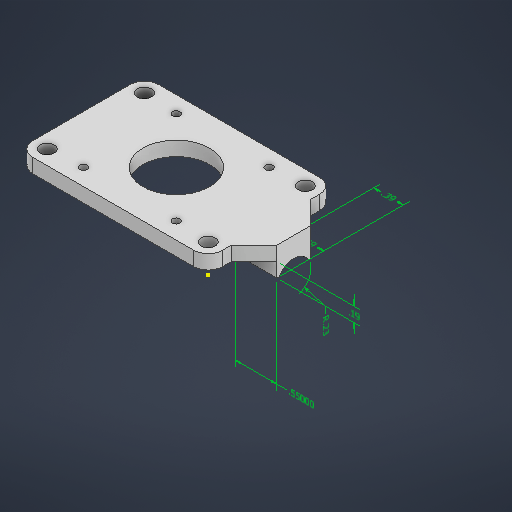
# Autodesk Inventor part: MotorTop
Saved by Autodesk Inventor 2026 (Build 300175000, 175)
## iProperties
Created: 2025-04-10
Part Number: MotorTop
Material: Generic
Document SubType Name: Modeling
Designer: jjgen
Density: 1 g/cm^3
Appearance: Default
Author: jjgen
## iProperties of the stored document MotorTop_3DPrint.ipt
Created: 2025-04-17
Part Number: MotorTop_3DPrint
Material: Generic
Document SubType Name: Modeling
Designer: sdcel
Density: 1 g/cm^3
Appearance: Default
Author: sdcel
Autodesk Inventor part; units mm, degrees
ref_plane "YZ Plane" through (0, 0, 0) normal (1, 0, 0) x (0, 1, 0)
ref_plane "XZ Plane" through (0, 0, 0) normal (0, 1, 0) x (-1, 0, 0)
ref_plane "XY Plane" through (0, 0, 0) normal (0, 0, 1) x (1, 0, 0)
sketch "Sketch1" plane through (0, 0, 0) normal (0, 1, 0) x (-1, 0, 0)
  line L0 (0, -4.826) -> (0, -37.338)
  line L1 (4.826, -42.164) -> (58.674, -42.164)
  line L2 (63.5, -37.338) -> (63.5, -4.826)
  line L3 (58.674, 0) -> (4.826, 0)
  arc A0 (4.826, 0) -> (0, -4.826) centre (4.826, -4.826) ccw
  arc A1 (63.5, -4.826) -> (58.674, 0) centre (58.674, -4.826) ccw
  arc A2 (58.674, -42.164) -> (63.5, -37.338) centre (58.674, -37.338) ccw
  arc A3 (0, -37.338) -> (4.826, -42.164) centre (4.826, -37.338) ccw
  circle A4 centre (4.826, -4.826) radius 4.826
  circle A5 centre (4.826, -37.338) radius 4.826
  circle A6 centre (58.674, -37.338) radius 4.826
  circle A7 centre (58.674, -4.826) radius 4.826
  circle A8 centre (58.674, -4.826) radius 2.3812
  circle A9 centre (58.674, -37.338) radius 2.3812
  circle A10 centre (4.826, -37.338) radius 2.3812
  circle A11 centre (4.826, -4.826) radius 2.3813
  point P0 (0, 0)
  point P1 (0, -42.164)
  point P2 (63.5, -42.164)
  dimension "d0" = 42.164
  dimension "d1" = 63.5
  dimension "d2" = 4.826
  dimension "d3" = 4.7625
  dimension "d4" = 4.7625
  dimension "d5" = 4.7625
  constraints: 10 centre point, 8 coincident, 8 end point, 8 point on circle, 8 tangent, 6 point on line, 5 equal radius, 3 perpendicular, 2 vertical alignment, 1 vertical, 4 other
  measures "d0" distance of point (0, 0) point (0, -42.164)
  measures "d1" distance of point (0, -42.164) point (63.5, -42.164)
  measures "d2" radius of A0
  measures "d3" diameter of A8
  measures "d4" diameter of A9
  measures "d5" diameter of A10
extrude "Extrusion1" add sketch "Sketch1" against normal blind 4.7625
sketch "Sketch2" plane through (0, -4.7625, 0) normal (0, -1, 0) x (1, 0, 0)
  line L0 (0, -37.338) -> (0, -4.826) projected
  line L1 (0, -21.082) -> (-63.5, -21.082)
  line L2 (-63.5, -4.826) -> (-63.5, -37.338) projected
  line L3 (-58.674, -42.164) -> (-4.826, -42.164) projected
  line L4 (-31.75, -42.164) -> (-31.75, 0)
  circle A0 centre (-31.75, -21.082) radius 11.176
  line L5 (-31.75, -21.082) -> (-16.2142, -5.5462)
  line L6 (-31.75, -21.082) -> (-9.779, -21.082) construction
  line L7 (-31.75, -21.082) -> (-47.2858, -5.5462)
  line L8 (-47.2858, -5.5462) -> (-31.75, -21.082)
  line L9 (-31.75, -21.082) -> (-47.2858, -36.6178)
  line L10 (-47.2858, -36.6178) -> (-31.75, -21.082)
  line L11 (-31.75, -21.082) -> (-16.2142, -36.6178)
  circle A1 centre (-16.2142, -5.5462) radius 1.27
  circle A2 centre (-16.2142, -36.6178) radius 1.27
  circle A3 centre (-47.2858, -36.6178) radius 1.27
  circle A4 centre (-47.2858, -5.5462) radius 1.27
  point P0 (0, 0)
  dimension "d8" = 22.352
  dimension "d9" = 21.971
  dimension "d10" = 45
  dimension "d11" = 21.971
  dimension "d12" = 21.971
  dimension "d13" = 2.54
  dimension "d14" = 2.54
  dimension "d15" = 2.54
  dimension "d16" = 2.54
  constraints: 18 end point, 5 centre point, 4 coincident, 4 midpoint, 2 collinear, 2 perpendicular, 1 equal length, 1 horizontal, 1 vertical
  measures "d8" diameter of A0
  measures "d9" distance of L5.start L5.end
  measures "d10" angle of L6 L5
  measures "d11" distance of L5.start L7.end
  measures "d12" distance of L5.start L9.end
  measures "d13" diameter of A1
  measures "d14" diameter of A2
  measures "d15" diameter of A3
  measures "d16" diameter of A4
extrude "Extrusion2" cut sketch "Sketch2" against normal blind 21.971
sketch "Sketch3" plane through (0, -4.7625, 0) normal (0, -1, 0) x (1, 0, 0)
  point P0 (0, 0)
sketch "Sketch4" plane through (0, 0, 0) normal (0, 1, 0) x (1, 0, 0)
  line L0 (0, 4.826) -> (0, 37.338) projected
  line L1 (0, 21.082) -> (0, 15.367)
  line L2 (0, 15.367) -> (0, 21.082)
  line L3 (0, 21.082) -> (0, 26.797)
  line L4 (0, 15.367) -> (7.62, 15.367)
  line L5 (7.62, 15.367) -> (7.62, 26.797)
  line L6 (7.62, 26.797) -> (0, 26.797)
  line L7 (7.62, 15.367) -> (0, 7.747)
  line L8 (7.62, 15.367) -> (18.3963, 15.367) construction
  line L9 (7.62, 26.797) -> (0, 34.417)
  line L10 (0, 15.367) -> (-6.35, 15.367)
  line L11 (-6.35, 15.367) -> (-6.35, 26.797)
  line L12 (-6.35, 26.797) -> (0, 26.797)
  point P0 (0, 0)
  dimension "d19" = 5.715
  dimension "d20" = 5.715
  dimension "d21" = 7.62
  dimension "d22" = 135
  dimension "d23" = 6.35
  constraints: 24 end point, 4 perpendicular, 4 point on line, 3 horizontal, 1 collinear, 1 equal length, 1 midpoint
  measures "d19" distance of L1.start L1.end
  measures "d20" distance of L1.start L3.end
  measures "d21" distance of L1.end L4.end
  measures "d22" angle of L7 L8
  measures "d23" distance of L1.end L10.end
extrude "Extrusion3" add sketch "Sketch4" against normal blind 4.7625 contours L0 L4 L7 | L6 L0 L9
extrude "Extrusion4" add sketch "Sketch4" against normal blind 9.525 contours L10 L11 L12 L0 | L0 L6 L5 L4
sketch "Sketch5" plane through (7.62, 0, -15.367) normal (1, 0, 0) x (0, 0, -1)
  line L0 (11.43, -4.7625) -> (0, -4.7625) projected
  line L1 (5.715, -4.7625) -> (5.715, -12.3825)
  circle A0 centre (5.715, -12.3825) radius 5.715
  point P0 (-15.367, 0)
  dimension "d28" = 7.62
  dimension "d29" = 11.43
  constraints: 2 end point, 1 centre point, 1 coincident, 1 midpoint, 1 vertical
  measures "d28" distance of L1.start L1.end
  measures "d29" diameter of A0
extrude "Extrusion5" cut sketch "Sketch5" against normal blind 9.9441
equation "\"d17\" = d9"
body "Solid1"
